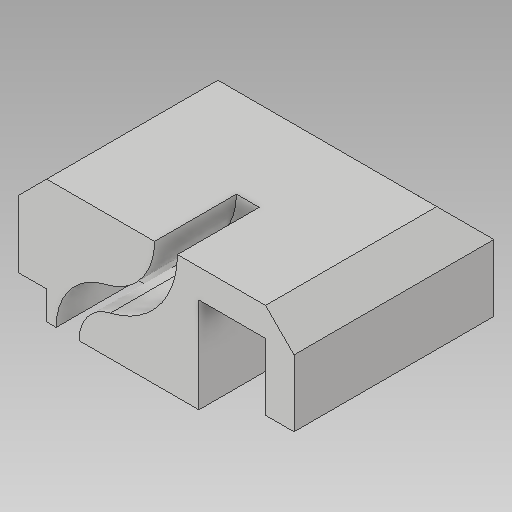
# Autodesk Inventor part: Dexter_hole_cover
Saved by Autodesk Inventor 2019.3 (Build 233278000, 278)
## iProperties
Created: 2019-04-07
Part Number: Dexter_hole_cover
Material: Generic
Document SubType Name: Modeling
Designer: Varga Daniel
Density: 1 g/cm^3
Appearance: Default
Author: Varga Daniel
Autodesk Inventor part; units mm, degrees
ref_plane "YZ Plane" through (0, 0, 0) normal (1, 0, 0) x (0, 1, 0)
ref_plane "XZ Plane" through (0, 0, 0) normal (0, 1, 0) x (-1, 0, 0)
ref_plane "XY Plane" through (0, 0, 0) normal (0, 0, 1) x (1, 0, 0)
ref_plane "Work Plane1" through (-0.8927, 0, 0) normal (0, 0, 1) x (1, 0, 0)
sketch "Sketch1" plane through (-0.8927, 0, 0) normal (0, 0, 1) x (1, 0, 0)
  line L0 (-11.5, 20) -> (-13, 20)
  line L1 (-13, 20) -> (-13, 23.5)
  line L2 (-13, 23.5) -> (-11.5, 25)
  line L3 (-11.5, 25) -> (0, 25)
  line L4 (0, 25) -> (1.5, 23.5)
  line L5 (1.5, 23.5) -> (1.5, 20)
  line L6 (1.5, 20) -> (0, 20)
  line L7 (-31.6913, 12.5) -> (-31.6913, 9.8) construction
  line L8 (-31.6913, 9.8) -> (-35.4978, 9.8) construction
  line L9 (-35.4978, 9.8) -> (-35.4978, 18.5) construction
  line L10 (-35.4978, 18.5) -> (-39.0518, 18.5) construction
  line L11 (-39.0518, 18.5) -> (-39.0518, 20) construction
  line L12 (-39.0518, 20) -> (-32.8955, 20) construction
  line L13 (-32.8955, 20) -> (-32.8955, 12.5) construction
  line L14 (-32.8955, 12.5) -> (-31.6913, 12.5) construction
  spline S0 degree 3 poles (-23.5617, 19.2) (-23.5277, 19.2) (-23.4877, 19.1924) (-23.4254, 19.1678) (-23.3919, 19.1467) (-23.3452, 19.1024) (-23.3234, 19.0717) (-23.2988, 19.0153) (-23.2913, 18.98) (-23.2913, 18.95) knots 0 0 0 0 0.264645 0.264645 0.521327 0.521327 0.766032 0.766032 1 1 1 1 construction
  line L15 (-23.2913, 18.95) -> (-23.2913, 16) construction
  arc A0 (-23.2913, 16) -> (-23.2913, 14) centre (-21, 15) ccw construction
  line L16 (-23.2913, 14) -> (-23.2913, 10.8) construction
  line L17 (-23.2913, 10.8) -> (-24.7, 10.8) construction
  line L18 (-24.7, 10.8) -> (-24.7, 18.5) construction
  line L19 (-24.7, 18.5) -> (-25.3022, 18.5) construction
  line L20 (-25.3022, 18.5) -> (-25.3022, 9.8) construction
  line L21 (-25.3022, 9.8) -> (-29.1087, 9.8) construction
  line L22 (-29.1087, 9.8) -> (-29.1087, 12.5) construction
  line L23 (-29.1087, 12.5) -> (-27.9045, 12.5) construction
  line L24 (-27.9045, 12.5) -> (-27.9045, 20) construction
  line L25 (-27.9045, 20) -> (-24.873, 20) construction
  line L26 (-24.873, 20) -> (-24.873, 19.2) construction
  line L27 (-24.873, 19.2) -> (-23.5617, 19.2) construction
  spline S1 degree 3 poles (-18.7087, 18.95) (-18.7087, 18.98) (-18.7012, 19.0153) (-18.6766, 19.0717) (-18.6548, 19.1024) (-18.6081, 19.1467) (-18.5746, 19.1678) (-18.5123, 19.1924) (-18.4723, 19.2) (-18.4383, 19.2) knots 0 0 0 0 0.23397 0.23397 0.478678 0.478678 0.735362 0.735362 1 1 1 1 construction
  line L28 (-18.4383, 19.2) -> (-17.127, 19.2) construction
  line L29 (-17.127, 19.2) -> (-17.127, 20) construction
  line L30 (-17.127, 20) -> (-11.5, 20) construction
  line L31 (-11.5, 20) -> (0, 20) construction
  line L32 (0, 20) -> (5.127, 20) construction
  line L33 (5.127, 20) -> (5.127, 19.2) construction
  line L34 (5.127, 19.2) -> (6.4383, 19.2) construction
  spline S2 degree 3 poles (6.4383, 19.2) (6.4723, 19.2) (6.5123, 19.1924) (6.5746, 19.1678) (6.6081, 19.1467) (6.6548, 19.1024) (6.6766, 19.0717) (6.7012, 19.0153) (6.7087, 18.98) (6.7087, 18.95) knots 0 0 0 0 0.264645 0.264645 0.521327 0.521327 0.766032 0.766032 1 1 1 1 construction
  line L35 (6.7087, 18.95) -> (6.7087, 16) construction
  arc A1 (6.7087, 16) -> (6.7087, 14) centre (9, 15) ccw construction
  line L36 (6.7087, 14) -> (6.7087, 10.8) construction
  line L37 (6.7087, 10.8) -> (5.3, 10.8) construction
  line L38 (5.3, 10.8) -> (5.3, 18.5) construction
  line L39 (5.3, 18.5) -> (0, 18.5) construction
  line L40 (0, 18.5) -> (-11.5, 18.5) construction
  line L41 (-11.5, 18.5) -> (-17.3, 18.5) construction
  line L42 (-17.3, 18.5) -> (-17.3, 10.8) construction
  line L43 (-17.3, 10.8) -> (-18.7087, 10.8) construction
  line L44 (-18.7087, 10.8) -> (-18.7087, 14) construction
  arc A2 (-18.7087, 14) -> (-18.7087, 16) centre (-21, 15) ccw construction
  line L45 (-18.7087, 16) -> (-18.7087, 18.95) construction
  line L46 (-11.5, 20) -> (-11.5, 18.5) construction
  line L47 (0, 18.5) -> (0, 20) construction
  line L48 (-74.6, 0) -> (-76, 0) construction
  line L49 (-76, 0) -> (-76, 19.8) construction
  arc A3 (-75.8, 20) -> (-76, 19.8) centre (-75.8, 19.8) ccw construction
  line L50 (-75.8, 20) -> (-74.873, 20) construction
  line L51 (-74.873, 20) -> (-74.873, 19.2) construction
  line L52 (-74.873, 19.2) -> (-73.5617, 19.2) construction
  spline S3 degree 3 poles (-73.5617, 19.2) (-73.5277, 19.2) (-73.4877, 19.1924) (-73.4254, 19.1678) (-73.3919, 19.1467) (-73.3452, 19.1024) (-73.3234, 19.0717) (-73.2988, 19.0153) (-73.2913, 18.98) (-73.2913, 18.95) knots 0 0 0 0 0.264645 0.264645 0.521327 0.521327 0.766032 0.766032 1 1 1 1 construction
  line L53 (-73.2913, 18.95) -> (-73.2913, 16) construction
  arc A4 (-73.2913, 16) -> (-73.2913, 14) centre (-71, 15) ccw construction
  line L54 (-73.2913, 14) -> (-73.2913, 10.8) construction
  line L55 (-73.2913, 10.8) -> (-74.6, 10.8) construction
  line L56 (-74.6, 10.8) -> (-74.6, 0) construction
  line L57 (12.6, 4.3589) -> (12.6, 10.8) construction
  line L58 (12.6, 10.8) -> (11.2913, 10.8) construction
  line L59 (11.2913, 10.8) -> (11.2913, 14) construction
  arc A5 (11.2913, 14) -> (11.2913, 16) centre (9, 15) ccw construction
  line L60 (11.2913, 16) -> (11.2913, 18.95) construction
  spline S4 degree 3 poles (11.2913, 18.95) (11.2913, 18.98) (11.2988, 19.0153) (11.3234, 19.0717) (11.3452, 19.1024) (11.3919, 19.1467) (11.4254, 19.1678) (11.4877, 19.1924) (11.5277, 19.2) (11.5617, 19.2) knots 0 0 0 0 0.23397 0.23397 0.478678 0.478678 0.735362 0.735362 1 1 1 1 construction
  line L61 (11.5617, 19.2) -> (12.873, 19.2) construction
  line L62 (12.873, 19.2) -> (12.873, 20) construction
  line L63 (12.873, 20) -> (13.8, 20) construction
  arc A6 (14, 19.8) -> (13.8, 20) centre (13.8, 19.8) ccw construction
  line L64 (14, 19.8) -> (14, 0) construction
  line L65 (14, 0) -> (13.1, 0) construction
  line L66 (13.1, 0) -> (13.1, 4.3589) construction
  line L67 (13.1, 4.3589) -> (12.6, 4.3589) construction
  line L68 (-62.0486, 18.4448) -> (-62.0486, 9.8) construction
  line L69 (-62.0486, 9.8) -> (-63.1468, 9.8) construction
  line L70 (-63.1468, 9.8) -> (-63.1468, 0) construction
  line L71 (-63.1468, 0) -> (-67.646, 0) construction
  line L72 (-67.646, 0) -> (-67.646, 10.8) construction
  line L73 (-67.646, 10.8) -> (-68.7087, 10.8) construction
  line L74 (-68.7087, 10.8) -> (-68.7087, 14) construction
  arc A7 (-68.7087, 14) -> (-68.7087, 16) centre (-71, 15) ccw construction
  line L75 (-68.7087, 16) -> (-68.7087, 18.95) construction
  spline S5 degree 3 poles (-68.7087, 18.95) (-68.7087, 18.98) (-68.7012, 19.0153) (-68.6766, 19.0717) (-68.6548, 19.1024) (-68.6081, 19.1467) (-68.5746, 19.1678) (-68.5123, 19.1924) (-68.4723, 19.2) (-68.4383, 19.2) knots 0 0 0 0 0.23397 0.23397 0.478678 0.478678 0.735362 0.735362 1 1 1 1 construction
  line L76 (-68.4383, 19.2) -> (-67.127, 19.2) construction
  line L77 (-67.127, 19.2) -> (-67.127, 20) construction
  line L78 (-67.127, 20) -> (-65.7077, 20) construction
  line L79 (-65.7077, 20) -> (-65.7077, 10) construction
  line L80 (-65.7077, 10) -> (-63.9869, 10) construction
  line L81 (-63.9869, 10) -> (-63.9869, 20) construction
  line L82 (-63.9869, 20) -> (-61.7482, 20) construction
  line L83 (-61.7482, 20) -> (-61.7482, 18.5) construction
  line L84 (-61.7482, 18.5) -> (-62.0482, 18.5) construction
  spline S6 degree 3 poles (-62.0482, 18.5) (-62.0483, 18.494) (-62.0483, 18.4879) (-62.0485, 18.4695) (-62.0486, 18.4572) (-62.0486, 18.4448) knots 0 0 0 0 0.32805 0.32805 1 1 1 1 construction
  line L85 (-11.5, 20) -> (-11.5, 18.5)
  line L86 (-3.5, 18.5) -> (-3.5, 20)
  line L87 (-3.5, 20) -> (-3.5, 23.5)
  line L88 (-3.5, 23.5) -> (0, 23.5)
  line L89 (0, 23.5) -> (0, 20)
  line L90 (-3.5, 20) -> (0, 20)
  line L91 (-3.5, 18.5) -> (-11.5, 18.5)
  line L92 (-3.5, 20) -> (-11.5, 20)
  point P0 (0.8927, 0)
  dimension "d0" = 1.5
  dimension "d1" = 1.5
  dimension "d2" = 3.5
  dimension "d3" = 3.5
  dimension "d4" = 135
  dimension "d5" = 135
  dimension "d6" = 1.5
  dimension "d10" = 1.5
  dimension "d11" = 3.5
  dimension "d12" = 3.5
  constraints: 186 end point, 40 vertical, 37 horizontal, 16 point on circle, 8 centre point, 5 perpendicular, 4 collinear, 3 parallel, 3 point on line, 1 coincident, 125 other
  measures "d0" distance of L0.start L0.end
  measures "d1" distance from line of L6.end L5
  measures "d2" distance of L4.end L5.end
  measures "d3" distance of L0.end L1.end
  measures "d4" angle of L2 L1
  measures "d5" angle of L4 L5
  measures "d6" distance from line of L4.end L3
  measures "d10" distance between parallel lines of L3 L88
  measures "d11" distance between parallel lines of L88 L31
  measures "d12" distance between parallel lines of L87 L89
extrude "Extrusion1" add sketch "Sketch1" along normal blind 9 contours L92 L86 L91 L85 | L0 L1 L2 L3 L4 L5 L6 L89 L88 L87 L92
extrude "Extrusion2" add sketch "Sketch1" against normal blind 1.5 contours L0 L1 L2 L3 L4 L5 L6 L89 L88 L87 L92 | L87 L88 L89 L90
chamfer "Chamfer1" distance 1.5 angle 45 1 edges at (-6.6427, 25, -1.5)
sketch "Sketch2" plane through (-0.8927, 0, 9) normal (0, 0, 1) x (1, 0, 0)
  line L0 (-11.5, 20) -> (-11.5, 18.5) projected
  line L1 (-11.5, 18.5) -> (-3.5, 18.5) projected
  line L2 (-3.5, 18.5) -> (-3.5, 23.5) projected
  line L3 (-3.5, 23.5) -> (0, 23.5) projected
  line L4 (0, 23.5) -> (0, 20) projected
  line L5 (0, 20) -> (1.5, 20) projected
  line L6 (1.5, 20) -> (1.5, 23.5) projected
  line L7 (1.5, 23.5) -> (0, 25) projected
  line L8 (0, 25) -> (-11.5, 25) projected
  line L9 (-11.5, 25) -> (-13, 23.5) projected
  line L10 (-13, 23.5) -> (-13, 20) projected
  line L11 (-13, 20) -> (-11.5, 20) projected
  line L12 (-11.5, 20) -> (-11.5, 18.5) projected
  arc A0 (-8.4144, 21.75) -> (-11, 18.5) centre (-7.6646, 18.5) ccw
  arc A1 (-8.4144, 21.75) -> (-5.8287, 25) centre (-9.1641, 25) ccw
  arc A2 (-8.1446, 20.5807) -> (-9.8, 18.5) centre (-7.6646, 18.5) ccw
  arc A3 (-8.1446, 20.5807) -> (-4.6287, 25) centre (-9.1641, 25) ccw
  line L13 (-9.8, 18.5) -> (-11, 18.5)
  line L14 (-11.5, 18.5) -> (-3.5, 18.5) projected
  line L15 (-5.8287, 25) -> (-4.6287, 25)
  point P0 (0.8927, 0)
  dimension "d22" = 3.25
  dimension "d23" = 6.5
  dimension "d24" = 0.5
  dimension "d25" = 1.2
  constraints: 8 point on circle, 4 centre point, 4 end point, 2 collinear, 2 line through centre, 1 equal radius, 1 point on line, 1 other
  measures "d22" distance from line of A0.start L8
  measures "d23" distance between parallel lines of L1 L8
  measures "d24" distance from line of L13.end L0
  measures "d25" radial gap between concentric circles of A0 A2
extrude "Extrusion3" cut sketch "Sketch2" against normal blind 4.3 contours A0 A1 L8 A3 A2 L1
equation "\"d1\" = d0"
equation "\"d3\" = d2"
equation "\"d5\" = d4"
equation "\"d22\" = 0.5 * d23"
body "Solid1"
